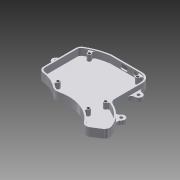
# Autodesk Inventor part: 20keyCaseLeft
Saved by Autodesk Inventor 2015 SP2 (Build 190223200, 223)
## iProperties
Created: 2015-12-14
Part Number: 20keyCaseLeft
Material: Aluminum 6061
Document SubType Name: Modeling
Designer: Josh
Density: 2.7 g/cm^3
Appearance: Aluminum - Flat
Author: Josh
Autodesk Inventor part; units mm, degrees
ref_plane "YZ Plane" through (0, 0, 0) normal (1, 0, 0) x (0, 1, 0)
ref_plane "XZ Plane" through (0, 0, 0) normal (0, 1, 0) x (-1, 0, 0)
ref_plane "XY Plane" through (0, 0, 0) normal (0, 0, 1) x (1, 0, 0)
sketch "Sketch1" plane through (0, 0, 0) normal (0, 0, 1) x (1, 0, 0)
  arc A0 (-26.3659, 13.35) -> (-32.6845, 7.6302) centre (-26.3659, 7) ccw projected
  arc A1 (-45.4912, -23.2226) -> (-32.6845, 7.6302) centre (-90.0314, 13.35) ccw projected
  arc A2 (-45.4912, -23.2226) -> (-48.0197, -34.2694) centre (-35.6761, -31.2819) ccw projected
  arc A3 (-72.5516, -103.5035) -> (-48.0197, -34.2694) centre (-113.3553, -50.0821) ccw projected
  arc A4 (-72.5516, -103.5035) -> (-74.0573, -111.9543) centre (-68.6971, -108.5498) ccw projected
  line L0 (-65.6044, -125.263) -> (-74.0573, -111.9543) projected
  arc A5 (-65.6044, -125.263) -> (-58.0785, -127.8278) centre (-60.2442, -121.8585) ccw projected
  arc A6 (-58.0785, -127.8278) -> (-25.4201, -97.1726) centre (-77.431, -74.4869) ccw projected
  arc A7 (-13.7792, -89.55) -> (-25.4201, -97.1726) centre (-13.7792, -102.25) ccw projected
  line L1 (46.6875, -50.0383) -> (46.6875, -25.2034)
  arc A8 (46.6208, -24.2852) -> (34.3306, 10.2569) centre (-46.1813, -37.8469) ccw projected
  arc A9 (34.3306, 10.2569) -> (28.8795, 13.35) centre (28.8795, 7) ccw projected
  line L2 (28.8795, 13.35) -> (-26.3659, 13.35) projected
  arc A10 (46.6875, -25.2034) -> (46.6208, -24.2852) centre (40.3375, -25.2034) ccw projected
  arc A11 (46.6875, -50.0383) -> (46.6913, -50.258) centre (53.0375, -50.0383) ccw projected
  arc A12 (37.0562, 11.8854) -> (28.8795, 16.525) centre (28.8795, 7) ccw
  arc A13 (49.7624, -23.8261) -> (37.0562, 11.8854) centre (-46.1813, -37.8469) ccw
  arc A14 (33.9875, -92.725) -> (49.8625, -76.85) centre (33.9875, -76.85) ccw
  arc A15 (-13.7792, -92.725) -> (-22.5099, -98.4419) centre (-13.7792, -102.25) ccw
  arc A16 (-56.9956, -130.8124) -> (-22.5099, -98.4419) centre (-77.431, -74.4869) ccw
  arc A17 (-68.2845, -126.9653) -> (-56.9956, -130.8124) centre (-60.2442, -121.8585) ccw
  arc A18 (-74.4788, -100.9803) -> (-76.7374, -113.6566) centre (-68.6971, -108.5498) ccw
  arc A19 (-74.4788, -100.9803) -> (-51.1056, -35.0162) centre (-113.3553, -50.0821) ccw
  arc A20 (-47.945, -21.2077) -> (-51.1056, -35.0162) centre (-35.6761, -31.2819) ccw
  arc A21 (-47.945, -21.2077) -> (-35.8439, 7.9453) centre (-90.0314, 13.35) ccw
  arc A22 (-26.3659, 16.525) -> (-35.8439, 7.9453) centre (-26.3659, 7) ccw
  line L3 (28.8795, 7) -> (41.1547, 14.3341)
  line L4 (28.8795, 7) -> (28.8795, 19.5487)
  line L5 (40.3375, -25.2034) -> (57.4912, -22.6966)
  line L6 (33.9875, -76.85) -> (54.188, -76.85)
  line L7 (33.9875, -76.85) -> (33.9875, -96.0222)
  line L8 (-13.7792, -102.25) -> (-13.7792, -82.4784)
  line L9 (-13.7792, -102.25) -> (-30.7157, -94.8628)
  line L10 (-60.2442, -121.8585) -> (-56.2126, -132.9705)
  line L11 (-60.2442, -121.8585) -> (-70.3002, -128.2456)
  line L12 (-68.6971, -108.5498) -> (-79.7497, -115.5698)
  line L13 (-68.6971, -108.5498) -> (-76.044, -98.9311)
  line L14 (-35.6761, -31.2819) -> (-55.7588, -36.1424)
  line L15 (-35.6761, -31.2819) -> (-51.2441, -18.4988)
  line L16 (-26.3659, 7) -> (-37.5753, 8.118)
  line L17 (-26.3659, 7) -> (-26.3659, 19.0257)
  line L18 (-68.2845, -126.9653) -> (-76.7374, -113.6566)
  line L19 (28.8795, 16.525) -> (-26.3659, 16.525)
  line L20 (33.9875, -92.725) -> (-13.7792, -92.725)
  arc A23 (49.8625, -25.2034) -> (49.7624, -23.8261) centre (40.3375, -25.2034) ccw
  line L21 (40.3375, -25.2034) -> (58.5046, -25.2034)
  line L22 (49.8625, -25.2034) -> (49.8625, -76.85)
  circle A24 centre (-12.1917, -91.1375) radius 1.5875
  line L23 (46.6875, -76.85) -> (46.6875, -25.2034) projected
  arc A25 (33.9875, -89.55) -> (46.6875, -76.85) centre (33.9875, -76.85) ccw projected
  line L24 (-13.7792, -89.55) -> (33.9875, -89.55)
  point P0 (0, 0)
  point P1 (46.6708, -24.7431)
  dimension "d2" = 3.175
  constraints: 44 end point, 32 point on line, 25 point on circle, 13 centre point, 8 concentric, 4 coincident, 3 parallel, 3 tangent
  measures "d2" diameter of A24
extrude "Extrusion1" add sketch "Sketch1" against normal blind 14.2875 contours L17 L16 A0 | L17 L19 L4 L2 | L2 L4 L3 A8 L5 L21 L1 L23 L6 L7 L24 A7 A6 L10 L11 L0 L12 L13 A3 L14 L15 A1 L16 L17 | A0 L16 A22 L17 | A1 L15 A21 L16 | L4 A12 L3 A9 | A9 L3 L4 | L15 L14 A2 | A2 L14 A20 L15 | L3 A13 L5 A8 | A3 L13 A19 L14 | L5 A23 L21 A10 | A10 L21 L5 | L13 L12 A4 | A4 L12 A18 L13 | L21 L22 L6 L23 L1 | L0 L11 L18 L12 | L11 L10 A5 | A5 L10 A17 L11 | A25 L7 L6 | L6 A14 L7 A25 | A6 L9 A16 L10 | L7 L20 A24 L24 | A7 L8 A15 L9 | A24 | A24 L8 L24 | L20 L8 A24
shell "Shell1" thickness 2.54 removed faces 1 at (-4.4642, -54.4609, 0)
sketch "Sketch3" plane through (0, 0, -14.2875) normal (0, 0, -1) x (-1, 0, 0)
  arc A0 (5.0932, 22.875) -> (11.4432, 16.525) centre (11.4432, 22.875) ccw projected
  circle A1 centre (-1.2568, 22.875) radius 6.35 projected
  circle A2 centre (-1.2568, 22.875) radius 2.5527
  arc A3 (-13.9568, 16.525) -> (-7.6068, 22.875) centre (-13.9568, 22.875) ccw projected
  line L0 (26.3659, 16.525) -> (-28.8795, 16.525) projected
  circle A4 centre (-21.2875, -99.075) radius 6.35 projected
  arc A5 (-8.5875, -92.725) -> (-14.9375, -99.075) centre (-8.5875, -99.075) ccw projected
  circle A6 centre (-21.2875, -99.075) radius 2.5527
  arc A7 (-27.6375, -99.075) -> (-33.9875, -92.725) centre (-33.9875, -99.075) ccw projected
  arc A8 (23.8454, -112.954) -> (25.6319, -104.6038) centre (20.1423, -107.7955) ccw projected
  circle A9 centre (27.5485, -118.1124) radius 6.35 projected
  circle A10 centre (27.5485, -118.1124) radius 2.5527
  arc A11 (40.6814, -121.8117) -> (32.1676, -122.4697) centre (36.7867, -126.8271) ccw projected
  arc A12 (22.5099, -98.4419) -> (56.9956, -130.8124) centre (77.431, -74.4869) ccw projected
  line L1 (-33.9875, -92.725) -> (13.7792, -92.725) projected
  arc A13 (5.0932, 22.875) -> (11.4432, 16.525) centre (11.4432, 22.875) ccw
  line L2 (-28.8795, 16.525) -> (26.3659, 16.525) projected
  arc A14 (-1.2568, 16.525) -> (5.0932, 22.875) centre (-1.2568, 22.875) ccw
  arc A15 (-13.9568, 16.525) -> (-7.6068, 22.875) centre (-13.9568, 22.875) ccw
  arc A16 (-7.6068, 22.875) -> (-1.2568, 16.525) centre (-1.2568, 22.875) ccw
  line L3 (11.4432, 16.525) -> (-13.9568, 16.525)
  line L4 (-1.2568, 16.525) -> (11.4432, 16.525)
  line L5 (-1.2568, 16.525) -> (-13.9568, 16.525)
  arc A17 (23.8454, -112.954) -> (25.6319, -104.6038) centre (20.1423, -107.7955) ccw
  arc A18 (40.6814, -121.8117) -> (32.1676, -122.4697) centre (36.7867, -126.8271) ccw
  arc A19 (32.1676, -122.4697) -> (32.3284, -113.9321) centre (27.5485, -118.1124) ccw
  arc A20 (32.3284, -113.9321) -> (23.8454, -112.954) centre (27.5485, -118.1124) ccw
  arc A21 (25.6319, -104.6038) -> (32.3284, -113.9321) centre (77.431, -74.4869) ccw
  arc A22 (32.3284, -113.9321) -> (40.6814, -121.8117) centre (77.431, -74.4869) ccw
  circle A23 centre (-1.2568, 22.875) radius 2.5527 projected
  circle A24 centre (-21.2875, -99.075) radius 2.5527 projected
  circle A25 centre (27.5485, -118.1124) radius 2.5527 projected
  point P0 (0, 0)
  constraints: 22 point on circle, 13 centre point, 11 concentric, 6 end point, 3 equal radius, 1 collinear, 1 horizontal alignment, 1 midpoint, 2 other
extrude "Extrusion3" add sketch "Sketch3" against normal blind 6.35
sketch "Sketch4" plane through (-26.3659, 13.985, -11.7475) normal (0, 0, 1) x (1, 0, 0)
  circle A0 centre (67.4089, -91.6238) radius 3.175
  circle A1 centre (60.5565, -15.386) radius 3.175
  circle A2 centre (-7.6486, -29.7847) radius 3.175
  circle A3 centre (-21.5918, -95.9142) radius 3.175
  circle A4 centre (3.2457, -100.6477) radius 3.175
  arc A5 (60.3534, -103.535) -> (73.0534, -90.835) centre (60.3534, -90.835) ccw projected
  circle A6 centre (71.5012, -93.3593) radius 1.27
  circle A7 centre (71.7834, -90.835) radius 1.27
  line L0 (58.9596, -83.185) -> (46.1596, -97.185)
  line L1 (58.9596, -97.185) -> (46.1596, -83.185)
  line L2 (44.5596, -82.185) -> (60.5596, -82.185)
  line L3 (60.5596, -82.185) -> (60.5596, -98.185)
  line L4 (60.5596, -98.185) -> (44.5596, -98.185)
  line L5 (44.5596, -98.185) -> (44.5596, -82.185)
  line L6 (44.5596, -82.185) -> (60.5596, -98.185) construction
  line L7 (60.5596, -82.185) -> (44.5596, -98.185) construction
  line L8 (73.0534, -39.1884) -> (73.0534, -90.835) projected
  circle A8 centre (63.9115, -12.4702) radius 1.27
  circle A9 centre (64.9605, -14.7834) radius 1.27
  circle A10 centre (-10.8411, -26.6918) radius 1.27
  circle A11 centre (-12.0136, -28.945) radius 1.27
  circle A12 centre (4.346, -104.9544) radius 1.27
  circle A13 centre (6.5247, -103.6488) radius 1.27
  circle A14 centre (-24.8655, -92.9074) radius 1.27
  circle A15 centre (-25.9776, -95.191) radius 1.27
  arc A16 (72.9867, -38.2702) -> (60.6965, -3.7281) centre (-19.8154, -51.8319) ccw projected
  arc A17 (73.6884, -39.1884) -> (73.615, -38.1784) centre (66.7034, -39.1884) ccw projected
  arc A18 (73.0534, -39.1884) -> (72.9867, -38.2702) centre (66.7034, -39.1884) ccw projected
  arc A19 (-19.6161, -36.8046) -> (-22.271, -48.4038) centre (-9.3102, -45.2669) ccw projected
  arc A20 (-19.6161, -36.8046) -> (-6.9505, -6.2918) centre (-63.6656, -0.635) ccw projected
  arc A21 (-46.5711, -116.9838) -> (-22.271, -48.4038) centre (-86.9894, -64.0671) ccw projected
  arc A22 (12.5867, -104.17) -> (1.5278, -111.4114) centre (12.5867, -116.235) ccw projected
  line L9 (60.3534, -104.17) -> (12.5867, -104.17) projected
  arc A23 (12.5867, -103.535) -> (0.9458, -111.1576) centre (12.5867, -116.235) ccw projected
  arc A24 (-31.7126, -141.8128) -> (0.9458, -111.1576) centre (-51.0651, -88.4719) ccw projected
  line L10 (60.3534, -103.535) -> (12.5867, -103.535) projected
  arc A25 (-19.1253, -37.2076) -> (-6.3186, -6.3548) centre (-63.6656, -0.635) ccw projected
  arc A26 (-19.1253, -37.2076) -> (-21.6538, -48.2544) centre (-9.3102, -45.2669) ccw projected
  arc A27 (-46.1857, -117.4885) -> (-21.6538, -48.2544) centre (-86.9894, -64.0671) ccw projected
  line L11 (61.3409, -25.235) -> (60.5565, -15.386)
  line L12 (60.5565, -15.386) -> (52.4159, -20.985)
  line L13 (0.3159, -20.985) -> (-7.6486, -29.7847)
  line L14 (-7.6486, -29.7847) -> (-3.0271, -40.7168)
  line L15 (-15.4193, -96.3924) -> (-21.5918, -95.9142)
  line L16 (-21.5918, -95.9142) -> (-17.8788, -100.8682)
  line L17 (7.4596, -97.185) -> (3.2457, -100.6477)
  line L18 (3.2457, -100.6477) -> (-2.1974, -100.9949)
  line L19 (20.8596, -83.185) -> (8.0596, -97.185)
  line L20 (20.8596, -97.185) -> (8.0596, -83.185)
  line L21 (1.8384, -87.5758) -> (-14.8526, -96.5897)
  line L22 (-2.7641, -100.7976) -> (-10.2502, -83.3678)
  line L23 (-11.4325, -81.8974) -> (-16.6924, -97.0081)
  line L24 (-16.6924, -97.0081) -> (-1.5818, -102.2681)
  line L25 (-1.5818, -102.2681) -> (3.6782, -87.1574)
  line L26 (3.6782, -87.1574) -> (-11.4325, -81.8974)
  line L27 (-11.4325, -81.8974) -> (-1.5818, -102.2681) construction
  line L28 (-16.6924, -97.0081) -> (3.6782, -87.1574) construction
  line L29 (6.4596, -82.185) -> (6.4596, -98.185)
  line L30 (6.4596, -98.185) -> (22.4596, -98.185)
  line L31 (22.4596, -98.185) -> (22.4596, -82.185)
  line L32 (22.4596, -82.185) -> (6.4596, -82.185)
  line L33 (6.4596, -82.185) -> (22.4596, -98.185) construction
  line L34 (6.4596, -98.185) -> (22.4596, -82.185) construction
  line L35 (21.4596, -83.185) -> (21.4596, -97.185) projected
  line L36 (2.405, -87.773) -> (-2.1974, -100.9949) projected
  arc A28 (60.3534, -104.17) -> (73.6884, -90.835) centre (60.3534, -90.835) ccw projected
  line L37 (73.6884, -39.1884) -> (73.6884, -90.835) projected
  arc A29 (68.9612, -88.8541) -> (73.6884, -86.0844) centre (70.5134, -86.0844) ccw
  arc A30 (69.845, -100.2015) -> (67.497, -94.7976) centre (67.5851, -97.9714) ccw
  arc A31 (73.615, -38.1784) -> (61.2416, -3.4024) centre (-19.8154, -51.8319) ccw projected
  arc A32 (61.2416, -3.4024) -> (55.2453, 0) centre (55.2453, -6.985) ccw projected
  arc A33 (73.615, -38.1784) -> (61.2416, -3.4024) centre (-19.8154, -51.8319) ccw projected
  arc A34 (68.4428, -18.2738) -> (63.0158, -17.3941) centre (65.4751, -19.4022) ccw
  arc A35 (60.6663, -12.2129) -> (63.5803, -7.5508) centre (60.7761, -9.0398) ccw
  arc A36 (-19.6161, -36.8046) -> (-6.9505, -6.2918) centre (-63.6656, -0.635) ccw projected
  arc A37 (-10.9227, -22.2401) -> (-7.8166, -26.6142) centre (-7.9846, -23.4436) ccw
  arc A38 (-10.3416, -31.4665) -> (-15.7062, -31.4327) centre (-13.0346, -33.1483) ccw
  arc A39 (-46.5711, -116.9838) -> (-22.271, -48.4038) centre (-86.9894, -64.0671) ccw projected
  arc A40 (-24.2291, -97.6821) -> (-29.6027, -97.8396) centre (-26.8664, -99.4499) ccw
  arc A41 (-25.0157, -88.4203) -> (-21.8263, -92.7479) centre (-22.0607, -89.5815) ccw
  arc A42 (3.2878, -108.5477) -> (2.0432, -103.5862) centre (0.8407, -106.5247) ccw
  arc A43 (6.404, -100.9729) -> (10.1924, -104.41) centre (9.5623, -101.2981) ccw
  arc A44 (12.5867, -104.17) -> (1.5278, -111.4114) centre (12.5867, -116.235) ccw projected
  point P0 (26.3659, -13.985)
  point P1 (52.5596, -90.185)
  point P2 (-6.5071, -92.0827)
  point P3 (14.4596, -90.185)
  dimension "d10" = 6.35
  dimension "d11" = 2.54
  dimension "d12" = 16
  constraints: 64 end point, 45 point on circle, 35 equal radius, 28 tangent, 24 centre point, 9 equal length, 9 midpoint, 8 parallel, 3 perpendicular, 1 coincident, 1 horizontal, 1 horizontal alignment, 1 point on line, 27 other
  measures "d10" diameter of A0
  measures "d11" diameter of A6
  measures "d12" distance of L3.end L4.end
extrude "Extrusion4" add sketch "Sketch4" along normal blind 10.16 contours A0 | A29 L8 A7 A0 | A0 A6 A5 A30 | A7 A6 A0 | A7 | A29 L37 A28 A30 A5 L8 | A6 | A5 A6 A7 | A34 A1 A9 A16 | A16 A35 A31 A34 | A43 A22 A42 A23 | A23 A13 A43 | A9 | A9 A8 A16 | A1 L11 L12 | A23 A12 A13 | A13 A43 | A9 A1 A8 | A8 | A8 A1 A35 A16 | A1 L12 L11 | A12 A42 | A12 A4 A13 | A23 A42 A12 | A13 A4 A43 | A12 A42 A4 | A4 L18 L17 | A4 L17 L18 | A2 L14 L13 | L13 L14 A2 | A2 A10 A37 | A38 A11 A2 | A2 A11 A10 | A10 A37 | A11 A38 | A11 A25 A10 | A10 A25 A37 | A38 A25 A11 | A25 A38 A20 A37 | A41 A14 A27 | A27 A40 A21 A41 | A14 A41 | A14 A15 A27 | A14 A3 A15 | A15 A40 | A15 A40 A27 | A41 A3 A14 | A3 L15 L16 | A3 A40 A15 | A3 L16 L15 picked at (6.5217, -103.5877) picked at (4.3267, -104.9914) picked at (-10.606, -26.4374) picked at (-12.087, -29.2835) picked at (-25.2423, -93.1724) picked at (-26.0013, -94.7309)
sketch "Sketch5" plane through (-26.3659, 13.985, -1.5875) normal (0, 0, 1) x (1, 0, 0)
  arc A0 (60.6663, -12.2129) -> (63.0158, -17.3941) centre (60.5565, -15.386) ccw projected
  arc A1 (-10.3416, -31.4665) -> (-7.8166, -26.6142) centre (-7.6486, -29.7847) ccw projected
  arc A2 (-24.2291, -97.6821) -> (-21.8263, -92.7479) centre (-21.5918, -95.9142) ccw projected
  arc A3 (6.404, -100.9729) -> (2.0432, -103.5862) centre (3.2457, -100.6477) ccw projected
  arc A4 (68.9612, -88.8541) -> (67.497, -94.7976) centre (67.4089, -91.6238) ccw projected
  circle A5 centre (60.5565, -15.386) radius 2.0828
  circle A6 centre (67.4089, -91.6238) radius 2.0828
  circle A7 centre (3.2457, -100.6477) radius 2.0828
  circle A8 centre (-7.6486, -29.7847) radius 2.0828
  circle A9 centre (-21.5918, -95.9142) radius 2.0828
  point P0 (26.3659, -13.985)
  dimension "d15" = 4.1656
  constraints: 5 centre point, 5 coincident, 4 equal radius
  measures "d15" diameter of A6
extrude "Extrusion5" cut sketch "Sketch5" against normal blind 10.16
thread "Thread1" size "8-32 UNC" class "2B" standard "ANSI Unified Screw Threads" full length
thread "Thread2" size "8-32 UNC" class "2B" standard "ANSI Unified Screw Threads" full length
thread "Thread3" size "8-32 UNC" class "2B" standard "ANSI Unified Screw Threads" full length
thread "Thread4" size "8-32 UNC" class "2B" standard "ANSI Unified Screw Threads" full length
thread "Thread5" size "8-32 UNC" class "2B" standard "ANSI Unified Screw Threads" full length
sketch "Sketch6" plane through (49.8625, -76.85, 0) normal (1, 0, 0) x (0, 0, -1)
  line L0 (0, 0) -> (14.2875, 0) projected
  line L1 (14.2875, 51.6466) -> (14.2875, 0) projected
  line L2 (0, 51.6466) -> (14.2875, 51.6466) projected
  line L3 (0, 45.75) -> (0, 31.75) projected
  line L4 (0, 26.7) -> (0, 12.7) projected
  line L5 (0, 7.65) -> (0, -6.35) projected
  line L6 (11.7475, 2.4147) -> (11.7475, -1.9129) projected
  line L7 (11.7475, -1.9129) -> (11.7475, -6.8471) projected
  line L8 (11.7475, -6.8471) -> (11.7475, -7.0046) projected
  line L9 (11.7475, -26.1488) -> (11.7475, -7.0046) projected
  line L10 (11.7475, -35.4448) -> (11.7475, -26.1488) projected
  line L11 (11.7475, -48.7535) -> (11.7475, -35.4448) projected
  line L12 (11.7475, -51.5747) -> (11.7475, -48.7535) projected
  line L13 (11.7475, -20.5764) -> (11.7475, -51.5747) projected
  line L14 (11.7475, -17.7127) -> (11.7475, -20.5764) projected
  line L15 (11.7475, -17.7127) -> (11.7475, -12.7512) projected
  line L16 (11.7475, -12.7512) -> (11.7475, -10.1379) projected
  line L17 (11.7475, -10.1379) -> (11.7475, -13.575) projected
  line L18 (11.7475, -13.335) -> (11.7475, -13.575) projected
  line L19 (11.7475, -9.3665) -> (11.7475, -13.335) projected
  line L20 (11.7475, -9.3665) -> (11.7475, -3.9626) projected
  line L21 (11.7475, -3.9626) -> (11.7475, 1.9809) projected
  line L22 (11.7475, 1.9809) -> (11.7475, 4.7506) projected
  line L23 (11.7475, 51.6466) -> (11.7475, 4.7506) projected
  line L24 (11.7475, 52.6566) -> (11.7475, 51.6466) projected
  line L25 (11.7475, 72.5612) -> (11.7475, 52.6566) projected
  line L26 (11.7475, 72.5612) -> (11.7475, 73.4409) projected
  line L27 (11.7475, 73.4409) -> (11.7475, 78.6221) projected
  line L28 (11.7475, 78.6221) -> (11.7475, 83.2842) projected
  line L29 (11.7475, 87.4326) -> (11.7475, 83.2842) projected
  line L30 (11.7475, 90.835) -> (11.7475, 87.4326) projected
  line L31 (11.7475, 84.5432) -> (11.7475, 90.835) projected
  line L32 (11.7475, 68.5949) -> (11.7475, 84.5432) projected
  line L33 (11.7475, 68.5949) -> (11.7475, 64.2208) projected
  line L34 (11.7475, 64.2208) -> (11.7475, 59.3685) projected
  line L35 (11.7475, 59.3685) -> (11.7475, 59.4023) projected
  line L36 (11.7475, 54.0304) -> (11.7475, 59.4023) projected
  line L37 (11.7475, 42.4312) -> (11.7475, 54.0304) projected
  line L38 (11.7475, 2.4147) -> (11.7475, 42.4312) projected
  line L39 (1.397, 12.7) -> (1.397, 26.7) projected
  line L40 (1.397, 64.262) -> (1.397, -8.6428)
  line L41 (11.7475, 51.6466) -> (11.7475, 4.7506) projected
  line L42 (0, 31.75) -> (1.397, 31.75)
  line L43 (1.397, 31.75) -> (1.397, 26.7)
  line L44 (1.397, 26.7) -> (0, 26.7)
  line L45 (0, 26.7) -> (0, 31.75)
  line L46 (0, 12.7) -> (1.397, 12.7)
  line L47 (1.397, 12.7) -> (1.397, 7.65)
  line L48 (1.397, 7.65) -> (0, 7.65)
  line L49 (0, 7.65) -> (0, 12.7)
  line L50 (1.397, 31.75) -> (11.7475, 31.75)
  line L51 (11.7475, 31.75) -> (11.7475, 26.7)
  line L52 (11.7475, 26.7) -> (1.397, 26.7)
  line L53 (1.397, 26.7) -> (1.397, 31.75)
  line L54 (0, 12.7) -> (11.7475, 12.7)
  line L55 (11.7475, 12.7) -> (11.7475, 7.65)
  line L56 (11.7475, 7.65) -> (0, 7.65)
  line L57 (0, 7.65) -> (0, 12.7)
  line L58 (11.7475, 31.75) -> (1.397, 26.7)
  line L59 (11.7475, 26.7) -> (1.397, 31.75)
  line L60 (11.7475, 12.7) -> (1.397, 7.65)
  line L61 (11.7475, 7.65) -> (1.397, 12.7)
  circle A0 centre (6.5722, 10.175) radius 4.0005
  line L62 (10.3822, 33.9875) -> (2.7622, 33.9875)
  line L63 (2.7622, 33.9875) -> (2.7623, 24.4625)
  line L64 (2.7623, 24.4625) -> (10.3823, 24.4625)
  line L65 (10.3823, 24.4625) -> (10.3822, 33.9875)
  line L66 (10.3822, 33.9875) -> (2.7623, 24.4625) construction
  line L67 (2.7622, 33.9875) -> (10.3823, 24.4625) construction
  arc A1 (10.5184, 33.1938) -> (8.1372, 35.575) centre (8.1372, 33.1938) ccw
  arc A2 (5.0073, 35.575) -> (2.6261, 33.1938) centre (5.0073, 33.1938) ccw
  arc A3 (2.6261, 25.2563) -> (5.0073, 22.875) centre (5.0073, 25.2563) ccw
  arc A4 (8.1372, 22.875) -> (10.5184, 25.2563) centre (8.1372, 25.2563) ccw
  line L68 (10.5184, 33.1938) -> (10.5184, 25.2563)
  line L69 (8.1372, 35.575) -> (5.0073, 35.575)
  line L70 (2.6261, 33.1938) -> (2.6261, 25.2563)
  line L71 (5.0073, 22.875) -> (8.1372, 22.875)
  line L72 (0, 0) -> (0, 51.6466) projected
  line L73 (0, 35.575) -> (4.8326, 35.575)
  line L74 (4.8326, 35.575) -> (4.8326, 22.875)
  line L75 (4.8326, 22.875) -> (0, 22.875)
  line L76 (0, 22.875) -> (0, 35.575)
  line L77 (0, 35.575) -> (0.6985, 35.575)
  line L78 (0.6985, 35.575) -> (0.6985, 31.75)
  line L79 (0.6985, 31.75) -> (0, 31.75)
  line L80 (0, 31.75) -> (0, 35.575)
  line L81 (0, 22.875) -> (0.6985, 22.875)
  line L82 (0.6985, 22.875) -> (0.6985, 26.7)
  line L83 (0.6985, 26.7) -> (0, 26.7)
  line L84 (0, 26.7) -> (0, 22.875)
  point P0 (0, 76.85)
  point P1 (6.5722, 29.225)
  dimension "d28" = 8.001
  dimension "d29" = 7.62
  dimension "d30" = 9.525
  dimension "d31" = 2.3813
  dimension "d32" = 12.7
  constraints: 86 end point, 20 parallel, 11 point on circle, 9 perpendicular, 8 horizontal, 8 tangent, 6 midpoint, 5 centre point, 5 collinear, 5 point on line, 3 equal radius
  measures "d28" diameter of A0
  measures "d29" distance of L64.end L63.end
  measures "d30" distance of L64.end L62.start
  measures "d31" radius of A1
  measures "d32" distance of L73.end L74.end
sketch "Sketch8" plane through (49.8625, -76.85, 0) normal (1, 0, 0) x (0, 0, -1)
  line L0 (2.6261, 33.1938) -> (2.6261, 25.2563) projected
  arc A0 (5.0073, 35.575) -> (2.6261, 33.1938) centre (5.0073, 33.1938) ccw projected
  line L1 (8.1372, 35.575) -> (5.0073, 35.575) projected
  arc A1 (10.5184, 33.1938) -> (8.1372, 35.575) centre (8.1372, 33.1938) ccw projected
  line L2 (10.5184, 33.1938) -> (10.5184, 25.2563) projected
  arc A2 (8.1372, 22.875) -> (10.5184, 25.2563) centre (8.1372, 25.2563) ccw projected
  line L3 (5.0073, 22.875) -> (8.1372, 22.875) projected
  circle A3 centre (6.5722, 10.175) radius 4.0005 projected
  line L4 (0, 0) -> (0, 51.6466) projected
  line L5 (0, 0) -> (14.2875, 0) projected
  line L6 (14.2875, 51.6466) -> (14.2875, 0) projected
  line L7 (0, 51.6466) -> (14.2875, 51.6466) projected
  arc A4 (2.6261, 25.2563) -> (5.0073, 22.875) centre (5.0073, 25.2563) ccw projected
  point P0 (0, 76.85)
extrude "Extrusion7" cut sketch "Sketch8" against normal blind 8.763 contours A0 L1 A1 L2 A2 L3 A4 L0 | A3
body "Solid1"
